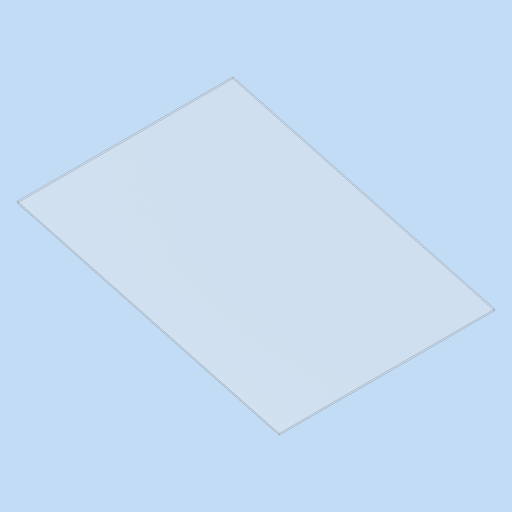
# Autodesk Inventor part: 부품2
Saved by Autodesk Inventor 2024.1 (Build 281209000, 209)
## iProperties
Created: 2024-01-19
Part Number: 부품2
Material: 아크릴
Document SubType Name: Modeling
Designer: KBU
Density: 1.188 g/cm^3
Appearance: 투명 - 선명
Author: KBU
Autodesk Inventor part; units mm, degrees
ref_plane "YZ Plane" through (0, 0, 0) normal (1, 0, 0) x (0, 1, 0)
ref_plane "XZ Plane" through (0, 0, 0) normal (0, 1, 0) x (-1, 0, 0)
ref_plane "XY Plane" through (0, 0, 0) normal (0, 0, 1) x (1, 0, 0)
sketch "스케치1" plane through (0, 0, 0) normal (0, 0, 1) x (1, 0, 0)
  line L0 (0, 0) -> (0, 5)
  line L1 (0, 0) -> (-850, 227.7568)
  line L2 (-12.9463, 0) -> (8.7754, 0)
  line L3 (0, 5) -> (-850, 232.7568)
  line L4 (-850, 227.7568) -> (-850, 232.7568)
  point P0 (-850, 230.2568)
  point P1 (-850, 242.7568)
  point P2 (0, 15)
  dimension "d0" = 15
  dimension "d1" = 5
  dimension "d2" = 850
  constraints: 10 end point, 2 point on line, 2 vertical, 1 coincident, 1 horizontal, 1 midpoint, 1 parallel
  measures "d0" angle of L1 L2
  measures "d1" distance of L0.start L0.end
  measures "d2" distance from line of L0 point (-850, 230.257)
extrude "돌출1" add sketch "스케치1" against normal blind 700
